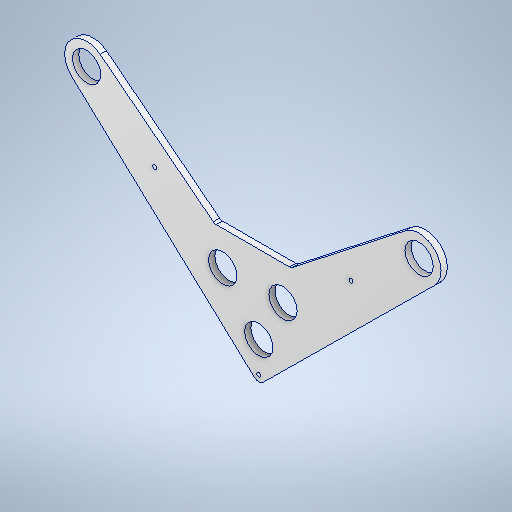
# Autodesk Inventor part: Gearbox #2 Plate
Saved by Autodesk Inventor 2025.1 (Build 291241020, 241B)
## iProperties
Created: 2024-09-19
Part Number: Gearbox #2 Plate
Material: Aluminum 6061
Document SubType Name: Modeling
Designer: xmand
Density: 2.7 g/cm^3
Appearance: Aluminum - Flat
Author: xmand
Autodesk Inventor part; units mm, degrees
ref_plane "YZ Plane" through (0, 0, 0) normal (1, 0, 0) x (0, 1, 0)
ref_plane "XZ Plane" through (0, 0, 0) normal (0, 1, 0) x (-1, 0, 0)
ref_plane "XY Plane" through (0, 0, 0) normal (0, 0, 1) x (1, 0, 0)
sketch "Sketch1" plane through (0, 0, 0) normal (0, 0, 1) x (1, 0, 0)
  circle A0 centre (0, 0) radius 20.32 construction
  circle A1 centre (0, 0) radius 22.86 construction
  circle A2 centre (24.5471, 44.4756) radius 30.48 construction
  circle A3 centre (-36.4129, 44.4756) radius 30.48 construction
  circle A4 centre (-36.4129, 44.4756) radius 33.02 construction
  line L0 (-15.4952, 18.9262) -> (-14.4815, 17.688)
  circle A5 centre (24.5471, 44.4756) radius 33.02 construction
  circle A6 centre (24.5471, 44.4756) radius 14.2875
  circle A7 centre (-36.4129, 44.4756) radius 14.2875
  circle A8 centre (0, 0) radius 14.2875
  circle A9 centre (24.5471, 44.4756) radius 19.1008 construction
  circle A10 centre (24.5471, 44.4756) radius 21.0058 construction
  circle A11 centre (-36.4129, 44.4756) radius 19.1008 construction
  circle A12 centre (-36.4129, 44.4756) radius 21.0058 construction
  line L1 (-36.4129, 44.4756) -> (-174.0993, 152.048) construction
  line L2 (24.5471, 44.4756) -> (162.2336, 152.048) construction
  circle A13 centre (-174.0993, 152.048) radius 14.2875
  circle A14 centre (162.2336, 152.048) radius 14.2875
  circle A15 centre (-174.0993, 152.048) radius 22.225 construction
  circle A16 centre (162.2336, 152.048) radius 22.225 construction
  line L3 (-160.4162, 169.5616) -> (-45.921, 80.1081)
  line L4 (-42.9811, 79.0958) -> (31.1154, 79.0958)
  arc A17 (31.1154, 79.0958) -> (34.0553, 80.1081) centre (31.1154, 83.871) ccw
  arc A18 (-45.921, 80.1081) -> (-42.9811, 79.0958) centre (-42.9811, 83.871) ccw
  line L5 (34.0553, 80.1081) -> (148.5505, 169.5616)
  line L6 (-36.4129, 79.0958) -> (-36.4129, 77.4956) construction
  arc A19 (177.8656, 136.2496) -> (148.5505, 169.5616) centre (162.2336, 152.048) ccw
  arc A20 (-160.4162, 169.5616) -> (-189.2001, 135.7411) centre (-174.0993, 152.048) ccw
  circle A21 centre (-105.2561, 98.2618) radius 2.0193
  circle A22 centre (0, -30.8102) radius 6.35 construction
  circle A23 centre (0, -30.8102) radius 2.0193
  line L7 (0, -22.86) -> (0, -24.4602)
  line L8 (-189.2001, 135.7411) -> (-4.3145, -35.4693)
  line L9 (177.8656, 136.2496) -> (4.4663, -35.324)
  arc A24 (-4.3145, -35.4693) -> (4.4663, -35.324) centre (0, -30.8102) ccw
  circle A25 centre (-105.2561, 98.2618) radius 6.35 construction
  circle A26 centre (93.3904, 98.2618) radius 6.35 construction
  circle A27 centre (93.3904, 98.2618) radius 2.0193
  circle A28 centre (-174.0993, 152.048) radius 50.8 construction
  circle A29 centre (162.2336, 152.048) radius 50.8 construction
  line L10 (-333.708, 192.5945) -> (-312.3217, 152.048) construction
  dimension "d0" = 40.64
  dimension "d3" = 2.54
  dimension "d9" = 60.96
  dimension "d10" = 2.54
  dimension "d12" = 1.6002
  dimension "d13" = 28.575
  dimension "d14" = 38.2016
  dimension "d15" = 42.0116
  dimension "d16" = 174.7266
  dimension "d17" = 104
  dimension "d18" = 28.575
  dimension "d24" = 44.45
  dimension "d25" = 44.45
  dimension "d37" = 4.7752
  dimension "d38" = 1.6002
  dimension "d39" = 4.0386
  dimension "d40" = 12.7
  dimension "d41" = 4.0386
  dimension "d42" = 1.6002
  dimension "d43" = 12.7
  dimension "d44" = 12.7
  dimension "d45" = 4.0386
  dimension "d46" = 87.3633
  dimension "d47" = 87.3633
  dimension "d48" = 101.6
  dimension "d49" = 101.6
  constraints: 30 centre point, 22 coincident, 22 end point, 21 point on circle, 16 tangent, 9 equal radius, 6 point on line, 2 horizontal alignment, 2 midpoint, 2 parallel, 2 vertical, 1 equal length, 1 horizontal
  measures "d0" diameter of A0
  measures "d3" radial gap between concentric circles of A1 A0
  measures "d9" diameter of A2
  measures "d10" radial gap between concentric circles of A3 A4
  measures "d12" distance of L0.start L0.end
  measures "d13" diameter of A6
  measures "d14" diameter of A9
  measures "d15" diameter of A10
  measures "d16" distance of L1.start L1.end
  measures "d17" angle of L2 L1
  measures "d18" diameter of A13
  measures "d24" diameter of A15
  measures "d25" diameter of A16
  measures "d37" radius of A18
  measures "d38" distance of L6.start L6.end
  measures "d39" diameter of A21
  measures "d40" diameter of A22
  measures "d41" diameter of A23
  measures "d42" distance of L7.start L7.end
  measures "d43" diameter of A25
  measures "d44" diameter of A26
  measures "d45" diameter of A27
  measures "d46" distance of A3.centre A21.centre
  measures "d47" distance of A26.centre A2.centre
  measures "d48" diameter of A29
  measures "d49" diameter of A28
extrude "Extrusion1" add sketch "Sketch1" along normal mid plane 6.35
body "Solid1"
